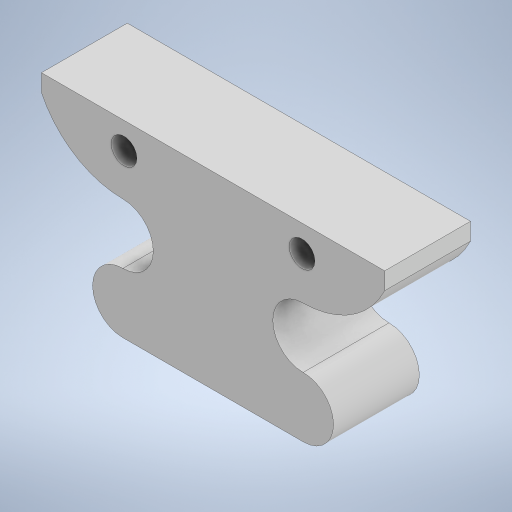
# Autodesk Inventor part: Zipperteethv5
Saved by Autodesk Inventor 2023.1 (Build 271208000, 208)
## iProperties
Created: 2022-11-01
Part Number: Zipperteethv5
Material: Generic
Document SubType Name: Modeling
Designer: Grimm
Density: 1 g/cm^3
Appearance: Default
Author: Grimm
Autodesk Inventor part; units mm, degrees
ref_plane "YZ Plane" through (0, 0, 0) normal (1, 0, 0) x (0, 1, 0)
ref_plane "XZ Plane" through (0, 0, 0) normal (0, 1, 0) x (-1, 0, 0)
ref_plane "XY Plane" through (0, 0, 0) normal (0, 0, 1) x (1, 0, 0)
sketch "Sketch1" plane through (0, 0, 0) normal (0, 0, 1) x (1, 0, 0)
  line L0 (-10.4625, 19.3656) -> (31.5375, 19.3656)
  line L1 (31.5375, 19.3656) -> (31.5375, -2.6344)
  line L2 (31.5375, -2.6344) -> (-10.4625, -2.6344)
  line L3 (-10.4625, -2.6344) -> (-10.4625, 19.3656)
  point P0 (0, 0)
  dimension "d0" = 42
  dimension "d1" = 22
  constraints: 8 end point, 2 parallel, 1 horizontal, 1 perpendicular
  measures "d0" distance of L1.end L2.end
  measures "d1" distance of L0.end L1.end
extrude "Extrusion1" add sketch "Sketch1" along normal blind 10
sketch "Sketch2" plane through (0, 0, 10) normal (0, 0, 1) x (1, 0, 0)
  line L0 (-10.4625, -2.6344) -> (31.5375, -2.6344) projected
  arc A0 (0.0751, -2.6344) -> (0.0375, 4.3656) centre (0.0751, 0.8657) ccw
  arc A1 (-0.0002, 11.3656) -> (0.0375, 4.3656) centre (-0.0002, 7.8655) ccw
  arc A2 (21.0375, 4.3656) -> (20.9998, -2.6344) centre (20.9998, 0.8657) ccw
  arc A3 (21.0375, 4.3656) -> (21.0751, 11.3656) centre (21.0751, 7.8655) ccw
  line L1 (-0.0002, 11.3656) -> (21.0751, 11.3656)
  line L2 (0.0751, 0.8657) -> (0.0375, 4.3656) construction
  line L3 (21.0751, 7.8655) -> (21.0375, 4.3656) construction
  line L4 (21.0375, 4.3656) -> (20.9998, 0.8657) construction
  line L5 (-10.4625, 19.3656) -> (-10.4625, -2.6344) projected
  line L6 (0.0375, 4.3656) -> (-0.0002, 7.8655) construction
  point P0 (0, 0)
  point P1 (10.5375, 11.3656)
  dimension "d4" = 21
  dimension "d5" = 21
  dimension "d6" = 14
  constraints: 10 end point, 9 point on circle, 6 tangent, 4 centre point, 3 equal radius, 2 point on line, 1 collinear, 1 horizontal, 1 midpoint
  measures "d4" distance of L3.end L2.end
  measures "d5" distance from line of L5 point (10.537, 11.366)
  measures "d6" distance between parallel lines of L0 L1
extrude "Extrusion2" cut sketch "Sketch2" against normal through all
sketch "Sketch3" plane through (0, 0, 10) normal (0, 0, 1) x (1, 0, 0)
  line L0 (-0.0002, 11.3656) -> (21.0751, 11.3656) projected
  arc A0 (-0.0002, 11.3656) -> (9.5375, 17.3656) centre (-0.0002, 21.9462) ccw
  arc A1 (11.5375, 17.3656) -> (21.0751, 11.3656) centre (21.0751, 21.9462) ccw
  line L1 (9.5375, 17.3656) -> (11.5375, 17.3656)
  line L2 (31.5375, 19.3656) -> (-10.4625, 19.3656) projected
  arc A2 (21.0375, 4.3656) -> (21.0751, 11.3656) centre (21.0751, 7.8655) ccw projected
  line L3 (-0.0002, 11.3656) -> (21.0751, 11.3656)
  point P0 (0, 0)
  dimension "d9" = 2
  dimension "d10" = 2
  constraints: 4 end point, 4 point on circle, 3 tangent, 2 centre point, 2 horizontal, 1 equal radius
  measures "d9" distance of L1.start L1.end
  measures "d10" distance between parallel lines of L1 L2
extrude "Extrusion3" cut sketch "Sketch3" against normal through all
pattern_linear "Rectangular Pattern1" count 2 spacing 42 along (-1, 0, 0) of "Extrusion1", "Extrusion2", "Extrusion3"
sketch "Sketch4" plane through (0, 0, 10) normal (0, 0, 1) x (1, 0, 0)
  line L0 (31.5375, 19.3656) -> (-52.4625, 19.3656) projected
  line L1 (-30.4543, 19.3656) -> (-30.4543, -2.6344)
  line L2 (-52.4625, -2.6344) -> (-41.9249, -2.6344) projected
  line L3 (-30.4543, -2.6344) -> (-52.4625, -2.6344)
  line L4 (-52.4625, -2.6344) -> (-52.4625, 19.3656)
  line L5 (-52.4625, 19.3656) -> (-30.4543, 19.3656)
  line L6 (9.5367, 19.3656) -> (9.5367, -2.6344)
  line L7 (20.9998, -2.6344) -> (31.5375, -2.6344) projected
  line L8 (9.5367, -2.6344) -> (31.5375, -2.6344)
  line L9 (31.5375, -2.6344) -> (31.5375, 19.3656)
  line L10 (31.5375, 19.3656) -> (9.5367, 19.3656)
  point P0 (0, 0)
  constraints: 16 end point, 6 perpendicular, 3 point on line, 2 collinear
extrude "Extrusion4" cut sketch "Sketch4" against normal through all
sketch "Sketch5" plane through (0, 0, 10) normal (0, 0, 1) x (1, 0, 0)
  arc A0 (-20.9625, 4.3656) -> (-20.9249, 11.3656) centre (-20.9249, 7.8655) ccw projected
  line L0 (-20.9625, 4.3656) -> (-21.1286, -11.0791) construction
  arc A1 (-0.0002, 11.3656) -> (0.0375, 4.3656) centre (-0.0002, 7.8655) ccw construction
  line L1 (-20.9625, 4.3656) -> (-9.8965, 4.2466) construction
  line L2 (-20.9625, 4.3656) -> (-20.6751, 31.0931) construction
  arc A2 (0.0751, -2.6344) -> (0.0375, 4.3656) centre (0.0751, 0.8657) ccw projected
  arc A3 (-20.9625, 4.3656) -> (-21.0002, -2.6344) centre (-21.0002, 0.8657) ccw projected
  line L3 (9.5367, 19.3656) -> (-30.4543, 19.3656) construction
  line L4 (-10.4588, 19.3656) -> (-10.4625, -2.6344) construction
  line L5 (-21.0002, -2.6344) -> (0.0751, -2.6344) construction
  line L6 (0.0375, 4.3656) -> (-2.5475, 4.3378) construction
  line L7 (0.0375, 4.3656) -> (0.6415, 4.3721) construction
  line L8 (0.0375, 4.3656) -> (-0.1492, 21.7223) construction
  point P0 (0, 0)
  point P1 (-20.8344, 16.2756)
  point P2 (-0.0906, 16.2766)
  constraints: 14 end point, 3 perpendicular, 3 point on line, 3 tangent, 2 midpoint
hole "Hole1" at (-20.8344, 16.2756, 10) at (-0.0906, 16.2766, 10) direction (0, 0, -1) diameter 3 end through all
body "Solid1"
